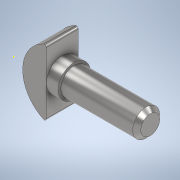
# Autodesk Inventor part: Tornillo
Saved by Autodesk Inventor 2021 (Build 250183000, 183)
## iProperties
Created: 2020-11-09
Part Number: Tornillo
Material: Acero inoxidable
Document SubType Name: Modeling
Designer: juanm
Density: 8 g/cm^3
Appearance: Semipulido
Author: juanm
Autodesk Inventor part; units mm, degrees
ref_plane "YZ Plane" through (0, 0, 0) normal (1, 0, 0) x (0, 1, 0)
ref_plane "XZ Plane" through (0, 0, 0) normal (0, 1, 0) x (-1, 0, 0)
ref_plane "XY Plane" through (0, 0, 0) normal (0, 0, 1) x (1, 0, 0)
sketch "Boceto1" plane through (0, 0, 0) normal (0, 0, 1) x (1, 0, 0)
  arc A0 (8.1351, 6.7837) -> (8.1351, -10.1182) centre (11.2305, -1.6673) ccw
  line L0 (8.1351, 6.7837) -> (8.1351, -10.1182)
  point P0 (0, 0)
  dimension "d2" = 18
  constraints: 2 end point, 2 point on circle, 1 centre point
  measures "d2" diameter of A0
extrude "Extrusión1" add sketch "Boceto1" along normal blind 8
fillet "Empalme3" radius 0.5 1 edges at (8.1351, 6.7837, 4)
fillet "Empalme4" radius 0.5 1 edges at (8.1351, -10.1182, 4)
sketch "Boceto4" plane through (8.1351, 6.0349, 8) normal (1, 0, 0) x (0, 0, -1)
  line L0 (8, 0.4531) -> (0, 0.4531) projected
  line L1 (4, 0.4531) -> (4, -7.7019)
  line L2 (0, -15.8574) -> (8, -15.8574) projected
  circle A0 centre (4, -7.7019) radius 4
  point P0 (8, -6.0349)
  dimension "d29" = 8.155
  dimension "d30" = 8
  constraints: 2 end point, 1 centre point, 1 coincident, 1 midpoint, 1 perpendicular
  measures "d29" distance of L1.start L1.end
  measures "d30" diameter of A0
extrude "Extrusión4" add sketch "Boceto4" along normal blind 3
sketch "Boceto5" plane through (11.1351, -1.6671, 4) normal (1, 0, 0) x (0, 0, -1)
  circle A0 centre (0, 0) radius 3.375
  point P0 (4, 1.6671)
  dimension "d33" = 6.75
  constraints: 1 centre point
  measures "d33" diameter of A0
extrude "Extrusión5" add sketch "Boceto5" along normal blind 19
chamfer "Chaflán2" distance 1 angle 45 1 edges at (30.1351, -1.6671, 7.375)
sketch "Boceto6" plane through (0, 0, 8) normal (0, 0, 1) x (1, 0, 0)
  point P0 (0, 0)
